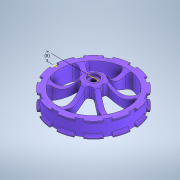
# Autodesk Inventor part: wheel_4
Saved by Autodesk Inventor 2020 (Build 240168000, 168)
## iProperties
Created: 2022-07-24
Part Number: wheel_4
Material: Типовые
Document SubType Name: Modeling
Designer: akapu
Density: 1 g/cm^3
Appearance: По умолчанию
Author: akapu
Autodesk Inventor part; units mm, degrees
ref_plane "YZ Plane" through (0, 0, 0) normal (1, 0, 0) x (0, 1, 0)
ref_plane "XZ Plane" through (0, 0, 0) normal (0, 1, 0) x (-1, 0, 0)
ref_plane "XY Plane" through (0, 0, 0) normal (0, 0, 1) x (1, 0, 0)
sketch "Эскиз1" plane through (0, 0, 0) normal (0, 1, 0) x (-1, 0, 0)
  circle A0 centre (0, 0) radius 34
  dimension "d0" = 68
  constraints: 1 centre point, 1 coincident
  measures "d0" diameter of A0
extrude "Выдавливание1" add sketch "Эскиз1" along normal blind 22
sketch "Эскиз2" plane through (0, 0, 0) normal (0, -1, 0) x (1, 0, 0)
  circle A0 centre (0, 0) radius 36
  dimension "d3" = 72
  constraints: 1 centre point, 1 coincident
  measures "d3" diameter of A0
sketch "Эскиз3" plane through (0, 0, 0) normal (0, -1, 0) x (1, 0, 0)
  point P0 (0, 0)
extrude "Выдавливание2" add sketch "Эскиз2" against normal blind 4
sketch "Эскиз4" plane through (0, 22, 0) normal (0, 1, 0) x (1, 0, 0)
  circle A0 centre (0, 0) radius 36
  dimension "d85" = 72
  constraints: 1 centre point, 1 coincident
  measures "d85" diameter of A0
extrude "Выдавливание3" add sketch "Эскиз4" against normal blind 12
sketch "Эскиз5" plane through (0, 0, 0) normal (0, -1, 0) x (1, 0, 0)
  line L0 (0, 0) -> (36, 0)
  circle A0 centre (0, 0) radius 36 projected
  line L1 (0, 0) -> (36, 0) construction
  line L2 (0, 0) -> (35.4531, -6.2513)
  line L3 (0, 0) -> (36, 0) construction
  circle A1 centre (0, 0) radius 36
  circle A2 centre (0, 0) radius 34
  line L4 (0, 0) -> (35.863, 3.1376)
  circle A3 centre (0, 0) radius 36 projected
  line L5 (0, 0) -> (36, 0) construction
  point P0 (34, 0)
  point P1 (33.8706, 2.9633)
  dimension "d9" = 10
  dimension "d65" = 5
  constraints: 12 end point, 4 horizontal, 3 point on circle, 2 coincident, 2 equal length, 1 centre point, 1 horizontal alignment, 2 other
  measures "d9" angle of L2 L3
  measures "d65" angle of L5 L4
extrude "Выдавливание4" cut sketch "Эскиз5" against normal blind 22 contours A2 L4 A0 L0
sketch "Эскиз6" plane through (34, 10, 0) normal (0, 0, 1) x (1, 0, 0)
  line L0 (0, -10) -> (0, -6) projected
  line L1 (2, -10) -> (0, -10) projected
  line L2 (2, -10) -> (0, -10)
  line L3 (0, -10) -> (0, -6)
  line L4 (-70, -10) -> (2, -10) projected
  line L5 (-70, 0) -> (2, 0) projected
  line L6 (2, 0) -> (0, 0)
  line L7 (0, 0) -> (0, 4)
  line L8 (0, 4) -> (2, 4)
  line L9 (2, 4) -> (2, 0)
  line L10 (-68, 0) -> (0, 0) projected
  line L11 (-34, -10) -> (-34, 12)
  line L12 (2, 12) -> (-70, 12) projected
  line L13 (2, -10) -> (0, -10)
  line L14 (0, -10) -> (0, -6)
  line L15 (0, -6) -> (2, -6)
  line L16 (2, -6) -> (2, -10)
  line L17 (2, 4) -> (2, 3.2)
  line L18 (2, -10) -> (2, -9.2)
  line L19 (2, -9.2) -> (0, -6)
  line L20 (1, -7.6) -> (0, -7.6)
  line L21 (2, 3.2) -> (0, 0)
  line L22 (1, 1.6) -> (0, 1.6)
  line L23 (2, -9.2) -> (0, -9.2)
  line L24 (0.5, -7.6) -> (0.5, -9.2)
  line L25 (2, 3.2) -> (0, 3.2)
  line L26 (0.5, 1.6) -> (0.5, 3.2)
  spline S0 degree 2 poles (2, 3.2) (-0.1925, 2.9189) (0, 0) knots 0 0 0 1 1 1
  spline S1 degree 2 poles (2, -9.2) (-0.1925, -8.9189) (0, -6) knots 0 0 0 1 1 1
  point P0 (1.4531, -10)
  point P1 (1.4531, 0)
  point P2 (-0.5165, 0)
  point P3 (1.4531, 12)
  point P4 (0.5, 2.4)
  point P5 (0.5, -8.4)
  point P6 (0, 0.8735)
  point P7 (0, -6.8735)
  dimension "d12" = 4
  dimension "d78" = 0.8
  dimension "d79" = 0.8
  constraints: 42 end point, 9 point on line, 8 perpendicular, 7 midpoint, 5 equal length, 2 horizontal, 6 other
  measures "d12" distance of L6.end L7.end
  measures "d78" distance of L8.end L17.end
  measures "d79" distance of L1.start L18.end
revolve "Вращение1" cut sketch "Эскиз6" angle 360 about axis through (0, 0, 0) along (0, 1, 0) contours L19 L15 L16 | S1 L24 L20 L19 | L0 L19 L20 S1 | L20 L24 S1 | L21 L9 L5 | L7 S0 L22 L21 | L22 L26 S0 L21 | S0 L26 L22
sketch "Эскиз8" plane through (0, 0, 0) normal (0, -1, 0) x (1, 0, 0)
  line L0 (0, 0) -> (6.1, 0)
  line L1 (6.1, -3.5218) -> (0, -7.0437)
  line L2 (0, -7.0437) -> (-6.1, -3.5218)
  line L3 (-6.1, -3.5218) -> (-6.1, 3.5218)
  line L4 (-6.1, 3.5218) -> (0, 7.0437)
  line L5 (0, 7.0437) -> (6.1, 3.5218)
  line L6 (6.1, 3.5218) -> (6.1, -3.5218)
  circle A0 centre (6.1, 3.5218) radius 0.5
  circle A1 centre (6.1, -3.5218) radius 0.5
  circle A2 centre (0, -7.0437) radius 0.5
  circle A3 centre (-6.1, -3.5218) radius 0.5
  circle A4 centre (-6.1, 3.5218) radius 0.5
  circle A5 centre (0, 7.0437) radius 0.5
  point P0 (-0.433, 6.7937)
  point P1 (-5.667, 3.7718)
  point P2 (-6.1, 3.0218)
  point P3 (-6.1, -3.0218)
  point P4 (-5.667, -3.7718)
  point P5 (-0.433, -6.7937)
  point P6 (0.433, -6.7937)
  point P7 (5.667, -3.7718)
  point P8 (6.1, -3.0218)
  point P9 (6.1, 3.0218)
  point P10 (5.667, 3.7718)
  point P11 (0.433, 6.7937)
  dimension "d16" = 6.1
  dimension "d17" = 1
  dimension "d18" = 1
  dimension "d19" = 1
  dimension "d20" = 1
  dimension "d21" = 1
  dimension "d22" = 1
  constraints: 14 end point, 7 coincident, 6 centre point, 1 horizontal, 1 midpoint, 13 other
  measures "d16" distance of L0.start L0.end
  measures "d17" diameter of A0
  measures "d18" diameter of A1
  measures "d19" diameter of A2
  measures "d20" diameter of A3
  measures "d21" diameter of A4
  measures "d22" diameter of A5
extrude "Выдавливание5" cut sketch "Эскиз8" against normal blind 17
sketch "Эскиз7" plane through (34, 22, 0) normal (0, 0, 1) x (1, 0, 0)
  line L0 (2, -8) -> (-70, -8) projected
  line L1 (2, -8) -> (-4, -8)
  line L2 (-4, -8) -> (-4, -22)
  line L3 (-70, -22) -> (2, -22) projected
  line L4 (2, 0) -> (-70, 0) projected
  line L5 (2, -8) -> (2, 0)
  line L6 (2, 0) -> (-34, 0)
  line L7 (-34, 0) -> (-34, -22)
  line L8 (-34, 0) -> (-25.5, 0)
  line L9 (-25.5, 0) -> (-25.5, -22)
  line L10 (-25.5, 0) -> (-4, -22)
  spline S0 degree 2 poles (-25.5, 0) (-16.4812, -17.446) (-4, -8) knots 0 0 0 1 1 1
  line L11 (-25.5, 0) -> (-25.5, -10)
  line L12 (0, -18) -> (-68, -18) projected
  spline S1 degree 2 poles (-25.5, -10) (-15.5868, -19.539) (-4, -22) knots 0 0 0 1 1 1
  line L13 (-25.5, -10) -> (-34, -10)
  line L14 (-25.5, -22) -> (-4, -22)
  line L15 (-34, -22) -> (-25.5, -22)
  point P0 (1.4531, -8)
  point P1 (1.4531, -22)
  point P2 (1.4531, 0)
  point P3 (-14.75, -11)
  point P4 (-14.75, -18)
  point P5 (-0.5165, -18)
  point P6 (-25.5, 0)
  dimension "d14" = 6
  dimension "d25" = 8.5
  dimension "d26" = 10
  constraints: 24 end point, 7 point on line, 5 perpendicular, 2 collinear, 1 midpoint, 1 vertical, 6 other
  measures "d14" distance of L0.start L1.end
  measures "d25" distance of L6.end L8.end
  measures "d26" distance of L8.end L11.end
revolve "Вращение2" cut sketch "Эскиз7" angle 360 about axis through (0, 22, 0) along (0, -1, 0) contours L0 L10 L4 L5 | S0 L10 L0 | L10 S0 L0 | L0 S0 L10 | L3 L9 L12 S1 | L3 L7 L12 L9 | L12 L9 S1 | L9 L12 L7 L13
fillet "Сопряжение1" radius 4 1 edges at (-8.5, 22, 0)
fillet "Сопряжение2" radius 4 1 edges at (-8.5, 12, 0)
sketch "Эскиз9" plane through (0, 12, 0) normal (0, -1, 0) x (1, 0, 0)
  circle A0 centre (0, 0) radius 8.5 projected
  circle A1 centre (0, 0) radius 30
  circle A2 centre (0, 0) radius 8.5
  circle A3 centre (0, 0) radius 30 projected
  line L0 (0, 8.5) -> (0, 30)
  line L1 (0, 0) -> (8.5, 0) construction
  line L2 (7.3612, 4.25) -> (25.9808, 15)
  line L3 (0, 8.5) -> (2, 8.5)
  line L4 (7.3612, 4.25) -> (6.3612, 5.9821)
  line L5 (7.3612, 4.25) -> (9.3612, 4.25) construction
  line L6 (7.9687, 6.9101) -> (21.9783, 14.9985)
  line L7 (6.3612, 5.9821) -> (6.1545, 5.8627)
  line L8 (2, 8.5) -> (2, 8.2614)
  line L9 (2, 10.3562) -> (2, 26.533)
  arc A4 (4.7812, 7.0278) -> (3.6957, 7.6546) centre (0, 0) ccw
  arc A5 (22.7536, 19.5518) -> (5.5556, 29.4811) centre (0, 0) ccw
  arc A6 (2, 10.3562) -> (3.6957, 7.6546) centre (5, 10.3562) ccw
  arc A7 (4.7812, 7.0278) -> (7.9687, 6.9101) centre (6.4687, 9.5082) ccw
  arc A8 (21.9783, 14.9985) -> (22.7536, 19.5518) centre (20.4783, 17.5966) ccw
  arc A9 (5.5556, 29.4811) -> (2, 26.533) centre (5, 26.533) ccw
  point P0 (24.923, 16.6987)
  point P1 (2, 29.9333)
  point P2 (2, 29.9333)
  point P3 (5.5556, 29.4811)
  point P4 (3.6957, 7.6546)
  point P5 (4.7812, 7.0278)
  dimension "d46" = 2
  dimension "d47" = 2
  dimension "d48" = 120
  dimension "d49" = 3
  constraints: 26 point on circle, 20 end point, 11 tangent, 8 centre point, 6 equal radius, 6 point on line, 3 horizontal, 2 coincident, 2 vertical, 1 equal length, 1 perpendicular
  measures "d46" distance of L0.start L3.end
  measures "d47" distance of L4.start L4.end
  measures "d48" angle of L5 L4
  measures "d49" radius of A6
extrude "Выдавливание6" cut sketch "Эскиз9" along normal mid plane 25 contours A0 A6 L9 A9 A1 A8 L6 A7
sketch "Эскиз10" plane through (0, 17, 0) normal (0, -1, 0) x (1, 0, 0)
  circle A0 centre (0, 0) radius 2.1
  dimension "d52" = 4.2
  constraints: 1 centre point, 1 coincident
  measures "d52" diameter of A0
extrude "Выдавливание7" cut sketch "Эскиз10" against normal blind 25
pattern_circular "Круговой массив1" count 6 over 360 about axis through (0, 17, 0) along (0, 1, 0) of "Выдавливание6"
sketch "Эскиз11" plane through (0, 0, 0) normal (0, -1, 0) x (1, 0, 0)
  arc A0 (35.863, 3.1376) -> (36, 0) centre (0, 0) ccw projected
  line L0 (0, 0) -> (36, 0) construction
  line L1 (0, 0) -> (36, 0)
  line L2 (36, 0) -> (34, 0) projected
  circle A1 centre (0, 0) radius 34
  circle A2 centre (0, 0) radius 36
  line L3 (0, 0) -> (35.863, -3.1376)
  arc A3 (35.863, 3.1376) -> (36, 0) centre (0, 0) ccw projected
  line L4 (0, 0) -> (36, 0) construction
  point P0 (35.4531, -6.2513)
  point P1 (35.4531, 6.2513)
  point P2 (36, 0)
  point P3 (33.8706, -2.9633)
  dimension "d64" = 5
  constraints: 8 end point, 3 point on circle, 2 coincident, 2 horizontal, 1 centre point, 1 collinear, 1 equal length, 3 other
  measures "d64" angle of L3 L4
extrude "Выдавливание8" cut sketch "Эскиз11" against normal blind 22 contours L3 A1 L1 A0
pattern_circular "Круговой массив2" count 12 over 360 about axis through (0, 17, 0) along (0, 1, 0) of "Выдавливание8", "Выдавливание4"
sketch "Эскиз13" plane through (6.1, 17, -3.0218) normal (-1, 0, 0) x (0, 0, 1)
  line L0 (7.0437, 0) -> (6.0437, 0) projected
  line L1 (-0.0138, -5) -> (0, -5) projected
  line L2 (6.0437, 0) -> (0, 0)
  line L3 (0, 0) -> (0, -5)
  line L4 (0, -5) -> (6.0437, -5)
  line L5 (6.0437, -5) -> (6.0437, 0)
  line L6 (6.0437, 0) -> (3.0218, 0)
  line L7 (0, 0) -> (-1, 0) projected
  line L8 (3.0218, 0) -> (0, 0)
  line L9 (0, 0) -> (1.5109, 0)
  line L10 (1.5109, 0) -> (1.5109, -5)
  line L11 (1.5109, -5) -> (1.6109, -5)
  line L12 (1.5109, 0) -> (1.7109, 0)
  line L13 (1.6109, -5) -> (1.7609, -5)
  line L14 (1.7109, 0) -> (1.8609, 0)
  line L15 (1.8609, 0) -> (1.7609, -5)
  point P0 (3.0218, -17)
  point P1 (6.7937, 0)
  point P2 (-0.75, 0)
  point P3 (1.8609, 0)
  point P4 (1.5109, 0)
  dimension "d66" = 0.1
  dimension "d67" = 0.2
  dimension "d68" = 0.15
  dimension "d69" = 0.15
  constraints: 26 end point, 5 point on line, 2 midpoint, 2 parallel, 2 perpendicular, 1 collinear, 1 horizontal
  measures "d66" distance of L10.end L11.end
  measures "d67" distance of L9.end L12.end
  measures "d68" distance of L11.end L13.end
  measures "d69" distance of L12.end L14.end
revolve "Вращение3" add sketch "Эскиз13" angle 360 about axis through (6.1, 17, -1.5109) along (0, -1, 0) contours L15 L4 L10 L2
sketch "Эскиз14" plane through (6.1, 12, 3.0218) normal (-1, 0, 0) x (0, 0, 1)
  line L0 (0, 0) -> (0.0138, 0) projected
  line L1 (-6.0437, 5) -> (-7.0437, 5) projected
  line L2 (0, 0) -> (-6.0437, 0)
  line L3 (-6.0437, 0) -> (-6.0437, 5)
  line L4 (-6.0437, 5) -> (0, 5)
  line L5 (0, 5) -> (0, 0)
  line L6 (1, 5) -> (0, 5) projected
  line L7 (0, 5) -> (-3.0218, 5)
  line L8 (-1.5109, 5) -> (-1.5109, 0)
  line L9 (-1.5109, 0) -> (-1.7609, 0)
  line L10 (-1.5109, 5) -> (-1.8609, 5)
  line L11 (-1.8609, 5) -> (-1.7609, 0)
  point P0 (-3.0218, -12)
  point P1 (-6.7937, 5)
  point P2 (0.75, 5)
  point P3 (-1.8609, 5)
  point P4 (-1.5109, 5)
  dimension "d71" = 0.25
  dimension "d72" = 0.35
  constraints: 18 end point, 3 point on line, 2 midpoint, 2 parallel, 2 perpendicular, 1 horizontal
  measures "d71" distance of L8.end L9.end
  measures "d72" distance of L8.start L10.end
revolve "Вращение4" add sketch "Эскиз14" angle 360 about axis through (6.1, 17, 1.5109) along (0, -1, 0) contours L2 L11 L4 L8
pattern_circular "Круговой массив3" count 6 over 360 about axis through (0, 17, 0) along (0, 1, 0) of "Вращение4", "Вращение3"
sketch "Эскиз15" plane through (0, 22, 0) normal (0, 1, 0) x (1, 0, 0)
  circle A0 centre (0, 0) radius 2.1 projected
  circle A1 centre (0, 0) radius 4.7
  dimension "d83" = 9.4
  constraints: 1 centre point, 1 coincident
  measures "d83" diameter of A1
extrude "Выдавливание9" cut sketch "Эскиз15" against normal blind 2
sketch "Эскиз16" plane through (0, 0, 0) normal (0, 0, 1) x (1, 0, 0)
  line L0 (-35.863, 14) -> (-32.6271, 14) projected
  line L1 (-4.7, 22) -> (4.7, 22) projected
  point P0 (0, 0)
  dimension "d84" = 8
  measures "d84" distance between parallel lines of L0 L1
